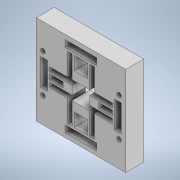
# Autodesk Inventor part: BearingFlexure
Saved by Autodesk Inventor 2022 (Build 260153000, 153)
## iProperties
Created: 2022-02-17
Part Number: BearingFlexure
Material: Generic
Document SubType Name: Modeling
Designer: 23ts01
Density: 1 g/cm^3
Appearance: Default
Author: 23ts01
Autodesk Inventor part; units mm, degrees
ref_plane "YZ Plane" through (0, 0, 0) normal (1, 0, 0) x (0, 1, 0)
ref_plane "XZ Plane" through (0, 0, 0) normal (0, 1, 0) x (-1, 0, 0)
ref_plane "XY Plane" through (0, 0, 0) normal (0, 0, 1) x (1, 0, 0)
sketch "Sketch1" plane through (0, 0, 0) normal (0, 0, 1) x (1, 0, 0)
  line L0 (0, 0) -> (127, 0)
  line L1 (127, 0) -> (127, 127)
  line L2 (127, 127) -> (0, 127)
  line L3 (0, 127) -> (0, 0)
  circle A0 centre (63.5, 63.5) radius 12.6844 construction
  circle A1 centre (9.4388, 90.7552) radius 3.175
  circle A2 centre (117.5612, 90.7552) radius 3.175
  circle A3 centre (117.5612, 36.2448) radius 3.175
  circle A4 centre (9.4388, 36.2448) radius 3.175
  line L4 (9.4388, 90.7552) -> (117.5612, 36.2448) construction
  line L5 (50.8, 50.8) -> (76.2, 50.8)
  line L6 (76.2, 50.8) -> (76.2, 76.2)
  line L7 (76.2, 76.2) -> (50.8, 76.2)
  line L8 (50.8, 76.2) -> (50.8, 50.8)
  line L9 (50.8, 50.8) -> (76.2, 76.2) construction
  line L10 (76.2, 50.8) -> (50.8, 76.2) construction
  point P0 (63.5, 127)
  point P1 (127, 63.5)
  dimension "d0" = 127
  dimension "d1" = 127
  dimension "d2" = 6.35
  dimension "d6" = 25.4
  dimension "d7" = 25.4
  constraints: 22 end point, 5 centre point, 5 midpoint, 4 parallel, 3 equal radius, 3 horizontal alignment, 3 vertical alignment, 2 horizontal, 2 perpendicular, 1 coincident
  measures "d0" distance of L0.end L1.end
  measures "d1" distance of L1.end L2.end
  measures "d2" diameter of A1
  measures "d6" distance of L6.end L7.end
  measures "d7" distance between parallel lines of L5 L7
extrude "Extrusion1" add sketch "Sketch1" along normal blind 25.4
sketch "Sketch2" plane through (0, 0, 25.4) normal (0, 0, 1) x (1, 0, 0)
  line L0 (50.8, 50.8) -> (50.8, 76.2) projected
  line L1 (19.05, 76.2) -> (50.8, 76.2)
  line L2 (50.8, 76.2) -> (50.8, 69.85)
  line L3 (50.8, 69.85) -> (19.05, 69.85)
  line L4 (19.05, 69.85) -> (19.05, 76.2)
  line L5 (19.05, 57.15) -> (50.8, 57.15)
  line L6 (50.8, 57.15) -> (50.8, 50.8)
  line L7 (50.8, 50.8) -> (19.05, 50.8)
  line L8 (19.05, 50.8) -> (19.05, 57.15)
  line L9 (19.05, 67.31) -> (38.1, 67.31)
  line L10 (38.1, 67.31) -> (38.1, 59.69)
  line L11 (38.1, 59.69) -> (19.05, 59.69)
  line L12 (19.05, 59.69) -> (19.05, 67.31)
  line L13 (50.8, 76.2) -> (76.2, 76.2) projected
  line L14 (0, 127) -> (0, 0) projected
  line L15 (127, 127) -> (0, 127) projected
  line L16 (63.5, 127) -> (63.5, 0) construction
  line L17 (0, 0) -> (127, 0) projected
  line L18 (76.2, 50.8) -> (76.2, 76.2)
  line L19 (107.95, 76.2) -> (76.2, 76.2)
  line L20 (76.2, 76.2) -> (76.2, 69.85)
  line L21 (76.2, 69.85) -> (107.95, 69.85)
  line L22 (107.95, 69.85) -> (107.95, 76.2)
  line L23 (107.95, 57.15) -> (76.2, 57.15)
  line L24 (76.2, 57.15) -> (76.2, 50.8)
  line L25 (76.2, 50.8) -> (107.95, 50.8)
  line L26 (107.95, 50.8) -> (107.95, 57.15)
  line L27 (107.95, 67.31) -> (88.9, 67.31)
  line L28 (88.9, 67.31) -> (88.9, 59.69)
  line L29 (88.9, 59.69) -> (107.95, 59.69)
  line L30 (107.95, 59.69) -> (107.95, 67.31)
  line L31 (127, 127) -> (127, 0)
  point P0 (50.8, 76.2)
  dimension "d8" = 6.35
  dimension "d9" = 6.35
  dimension "d10" = 2.54
  dimension "d11" = 2.54
  dimension "d12" = 12.7
  dimension "d13" = 19.05
  constraints: 54 end point, 13 symmetric about line, 6 parallel, 6 point on line, 3 horizontal, 3 perpendicular, 2 midpoint, 1 collinear
  measures "d8" distance between parallel lines of L1 L3
  measures "d9" distance between parallel lines of L5 L7
  measures "d10" distance between parallel lines of L11 L5
  measures "d11" distance between parallel lines of L3 L9
  measures "d12" distance between parallel lines of L0 L10
  measures "d13" distance between parallel lines of L14 L12
extrude "Extrusion2" cut sketch "Sketch2" against normal blind 25.4 contours L7 L8 L5 L0 | L23 L26 L25 L18 | L19 L22 L21 L18 | L3 L4 L1 L0 | L9 L10 L11 L12 | L30 L29 L28 L27
sketch "Sketch4" plane through (0, 0, 25.4) normal (0, 0, 1) x (1, 0, 0)
  line L0 (6.35, 82.55) -> (15.875, 82.55)
  line L1 (15.875, 82.55) -> (15.875, 44.45)
  line L2 (15.875, 44.45) -> (6.35, 44.45)
  line L3 (6.35, 44.45) -> (6.35, 82.55)
  line L4 (0, 127) -> (0, 0) projected
  line L5 (19.05, 69.85) -> (19.05, 76.2) projected
  line L6 (127, 127) -> (0, 127) projected
  line L7 (63.5, 127) -> (63.5, 0) construction
  line L8 (0, 0) -> (127, 0) projected
  line L9 (120.65, 82.55) -> (111.125, 82.55)
  line L10 (111.125, 82.55) -> (111.125, 44.45)
  line L11 (111.125, 44.45) -> (120.65, 44.45)
  line L12 (120.65, 44.45) -> (120.65, 82.55)
  line L13 (127, 127) -> (127, 0)
  line L14 (107.95, 69.85) -> (107.95, 76.2)
  point P0 (6.35, 63.5)
  point P1 (0, 63.5)
  point P2 (120.65, 63.5)
  dimension "d25" = 38.1
  dimension "d27" = 3.175
  dimension "d28" = 6.35
  constraints: 22 end point, 7 symmetric about line, 4 midpoint, 2 parallel, 1 horizontal, 1 horizontal alignment, 1 perpendicular
  measures "d25" distance between parallel lines of L0 L2
  measures "d27" distance between parallel lines of L5 L1
  measures "d28" distance between parallel lines of L4 L3
extrude "Extrusion4" cut sketch "Sketch4" against normal blind 25.4 contours L0 L1 L2 L3 | L12 L11 L10 L9
sketch "Sketch3" plane through (0, 0, 25.4) normal (0, 0, 1) x (1, 0, 0)
  line L0 (19.05, 50.8) -> (107.95, 50.8) projected
  line L1 (44.45, 50.8) -> (50.8, 50.8)
  line L2 (50.8, 50.8) -> (50.8, 19.05)
  line L3 (50.8, 19.05) -> (44.45, 19.05)
  line L4 (44.45, 19.05) -> (44.45, 50.8)
  line L5 (76.2, 50.8) -> (82.55, 50.8)
  line L6 (82.55, 50.8) -> (82.55, 19.05)
  line L7 (82.55, 19.05) -> (76.2, 19.05)
  line L8 (76.2, 19.05) -> (76.2, 50.8)
  line L9 (53.975, 38.1) -> (73.025, 38.1)
  line L10 (73.025, 38.1) -> (73.025, 19.05)
  line L11 (73.025, 19.05) -> (53.975, 19.05)
  line L12 (53.975, 19.05) -> (53.975, 38.1)
  line L13 (0, 0) -> (127, 0) projected
  line L14 (0, 127) -> (0, 0) projected
  line L15 (0, 63.5) -> (127, 63.5) construction
  line L16 (44.45, 76.2) -> (50.8, 76.2)
  line L17 (50.8, 76.2) -> (50.8, 107.95)
  line L18 (50.8, 107.95) -> (44.45, 107.95)
  line L19 (44.45, 107.95) -> (44.45, 76.2)
  line L20 (76.2, 76.2) -> (82.55, 76.2)
  line L21 (82.55, 76.2) -> (82.55, 107.95)
  line L22 (82.55, 107.95) -> (76.2, 107.95)
  line L23 (76.2, 107.95) -> (76.2, 76.2)
  line L24 (53.975, 88.9) -> (73.025, 88.9)
  line L25 (73.025, 88.9) -> (73.025, 107.95)
  line L26 (73.025, 107.95) -> (53.975, 107.95)
  line L27 (53.975, 107.95) -> (53.975, 88.9)
  point P0 (63.5, 19.05)
  point P1 (63.5, 50.8)
  point P2 (63.5, 107.95)
  point P3 (63.5, 76.2)
  dimension "d16" = 19.05
  dimension "d17" = 3.175
  dimension "d18" = 3.175
  dimension "d19" = 19.05
  dimension "d20" = 6.35
  dimension "d21" = 6.35
  dimension "d22" = 12.7
  constraints: 50 end point, 14 symmetric about line, 6 parallel, 6 point on line, 4 horizontal, 3 midpoint, 3 perpendicular, 1 vertical alignment
  measures "d16" distance between parallel lines of L10 L12
  measures "d17" distance between parallel lines of L8 L10
  measures "d18" distance between parallel lines of L12 L2
  measures "d19" distance between parallel lines of L11 L13
  measures "d20" distance between parallel lines of L2 L4
  measures "d21" distance between parallel lines of L6 L8
  measures "d22" distance from line of point (63.5, 50.8) L9
extrude "Extrusion3" cut sketch "Sketch3" against normal blind 25.4
sketch "Sketch5" plane through (0, 0, 25.4) normal (0, 0, 1) x (1, 0, 0)
  line L0 (41.275, 15.875) -> (85.725, 15.875)
  line L1 (85.725, 15.875) -> (85.725, 6.35)
  line L2 (85.725, 6.35) -> (41.275, 6.35)
  line L3 (41.275, 6.35) -> (41.275, 15.875)
  line L4 (0, 127) -> (0, 0) projected
  line L5 (0, 63.5) -> (127, 63.5) construction
  line L6 (127, 0) -> (127, 127) projected
  line L7 (73.025, 19.05) -> (53.975, 19.05) projected
  line L8 (0, 0) -> (127, 0) projected
  line L9 (41.275, 111.125) -> (85.725, 111.125)
  line L10 (85.725, 111.125) -> (85.725, 120.65)
  line L11 (85.725, 120.65) -> (41.275, 120.65)
  line L12 (41.275, 120.65) -> (41.275, 111.125)
  point P0 (63.5, 6.35)
  point P1 (63.5, 0)
  point P2 (63.5, 120.65)
  point P3 (63.5, 127)
  dimension "d31" = 3.175
  dimension "d32" = 6.35
  dimension "d33" = 44.45
  constraints: 18 end point, 6 symmetric about line, 4 midpoint, 2 parallel, 1 horizontal, 1 perpendicular, 1 vertical alignment
  measures "d31" distance between parallel lines of L7 L0
  measures "d32" distance between parallel lines of L2 L8
  measures "d33" distance between parallel lines of L1 L3
extrude "Extrusion5" cut sketch "Sketch5" against normal blind 25.4
body "Solid1"
